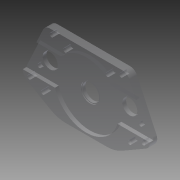
# Autodesk Inventor part: C11R1_ZP_middle wheel plate
Saved by Autodesk Inventor 2015 SP1 (Build 190203100, 203)
## iProperties
Created: 2016-01-16
Part Number: C11R1_ZP_middle wheel plate
Material: Polycarbonate, Clear
Document SubType Name: Modeling
Designer: Administrator
Density: 1.2 g/cm^3
Appearance: Polycarbonate - Clear
Mass: 206.575 g
Surface Area: 526.302 cm^2
Volume: 172.146 cm^3
Author: Administrator
Autodesk Inventor part; units mm, degrees
ref_plane "YZ Plane" through (0, 0, 0) normal (1, 0, 0) x (0, 1, 0)
ref_plane "XZ Plane" through (0, 0, 0) normal (0, 1, 0) x (-1, 0, 0)
sketch "Sketch1" plane through (0, 0, 0) normal (0, 0, 1) x (1, 0, 0)
  line L0 (0, 0) -> (0, 63.5)
  line L1 (0, 63.5) -> (203.2, 63.5)
  line L2 (203.2, 63.5) -> (203.2, 0)
  line L3 (0, 0) -> (203.2, 0)
  dimension "d0" = 63.5
  dimension "d1" = 203.2
  constraints: 8 end point, 2 perpendicular, 1 horizontal, 1 vertical
  measures "d0" distance of L0.start L0.end
  measures "d1" distance of L0.end L1.end
extrude "Extrusion1" add sketch "Sketch1" along normal blind 12.7
sketch "Sketch2" plane through (0, 0, 12.7) normal (0, 0, 1) x (1, 0, 0)
  line L0 (0, 63.5) -> (0, 0) projected
  line L1 (203.2, 0) -> (203.2, 63.5) projected
  line L2 (0, 57.2008) -> (203.2, 57.2008)
  line L3 (203.2, 57.2008) -> (203.2, 6.35)
  line L4 (203.2, 6.35) -> (0, 6.35)
  line L5 (0, 6.35) -> (0, 57.2008)
  line L6 (0, 63.5) -> (203.2, 63.5) projected
  line L7 (203.2, 0) -> (0, 0) projected
  dimension "d4" = 6.2992
  dimension "d5" = 6.35
  constraints: 8 end point, 2 parallel, 2 point on line, 1 horizontal, 1 perpendicular
  measures "d4" distance between parallel lines of L6 L2
  measures "d5" distance between parallel lines of L7 L4
extrude "Extrusion2" cut sketch "Sketch2" against normal blind 6.35 contours L2 L1 L4 L0
sketch "Sketch7" plane through (0, 0, 6.35) normal (0, 0, 1) x (1, 0, 0)
  line L0 (203.2, 6.35) -> (0, 6.35) projected
  line L1 (203.2, 57.2008) -> (203.2, 6.35) projected
  point P0 (0, 0)
  point P1 (101.6, 22.225)
  dimension "d19" = 15.875
  dimension "d20" = 101.6
  measures "d19" distance from line of L0 point (101.6, 22.225)
  measures "d20" distance from line of L1 point (101.6, 22.225)
hole "Hole1" at (101.6, 22.225, 6.35) direction (0, 0, -1) diameter 28.6258 end through all counterbore diameter 31.1658 counterbore depth 1.524
sketch "Sketch8" plane through (0, 0, 0) normal (0, 0, -1) x (-1, 0, 0)
  circle A0 centre (-34.2711, 35.4896) radius 17.78 projected
  circle A1 centre (-34.2711, 35.4896) radius 17.78 projected
  circle A2 centre (-34.2711, 35.4896) radius 17.78 projected
  line L0 (-203.2, 63.5) -> (-203.2, 0) projected
  point P0 (0, 0)
  point P1 (-168.9289, 35.4896)
  dimension "d28" = 34.2711
  measures "d28" distance from line of L0 point (-168.929, 35.49)
hole "Hole2" at (168.9289, 35.4896, 0) at (34.2711, 35.4896, 0) direction (0, 0, 1) diameter 25.4 end through all
sketch "Sketch10" plane through (0, 63.5, 0) normal (0, 1, 0) x (1, 0, 0)
  line L0 (0, -12.7) -> (203.2, -12.7)
  line L1 (203.2, -12.7) -> (203.2, 0)
  line L2 (203.2, 0) -> (0, 0)
  line L3 (0, 0) -> (0, -12.7)
  point P0 (0, 0)
  constraints: 8 end point, 2 parallel, 1 horizontal, 1 perpendicular
extrude "Extrusion5" add sketch "Sketch10" along normal blind 25.4
sketch "Sketch11" plane through (0, 6.35, 6.35) normal (-1, 0, 0) x (0, 0, 1)
  line L0 (0, 50.8508) -> (6.35, 50.8508) projected
  line L1 (6.35, 50.8508) -> (6.35, 82.55) projected
  line L2 (-6.35, 82.55) -> (6.35, 82.55) projected
  line L3 (-6.35, -6.35) -> (-6.35, 82.55) projected
  line L4 (6.35, 0) -> (6.35, -6.35) projected
  line L5 (6.35, 0) -> (0, 0) projected
  line L6 (0, 0) -> (0, 50.8508) projected
  line L7 (-6.35, -6.35) -> (6.35, -6.35) projected
extrude "Extrusion6" add sketch "Sketch11" along normal blind 9.525
sketch "Sketch12" plane through (203.2, 6.35, 6.35) normal (1, 0, 0) x (0, 0, -1)
  line L0 (-6.35, 50.8508) -> (0, 50.8508) projected
  line L1 (0, 50.8508) -> (0, 0) projected
  line L2 (0, 0) -> (-6.35, 0) projected
  line L3 (-6.35, -6.35) -> (-6.35, 0) projected
  line L4 (6.35, 82.55) -> (6.35, -6.35) projected
  line L5 (-6.35, 82.55) -> (6.35, 82.55) projected
  line L6 (-6.35, 50.8508) -> (-6.35, 82.55) projected
  line L7 (6.35, -6.35) -> (-6.35, -6.35) projected
extrude "Extrusion7" add sketch "Sketch12" along normal blind 9.525
sketch "Sketch15" plane through (0, 0, 0) normal (0, 0, -1) x (-1, 0, 0)
  circle A0 centre (-168.9289, 35.4896) radius 12.7 projected
  circle A1 centre (-34.2711, 35.4896) radius 12.7 projected
  circle A2 centre (-101.6, 22.225) radius 15.5829 projected
  line L0 (9.525, 57.2008) -> (-212.725, 57.2008) projected
  line L1 (9.525, 6.35) -> (9.525, 57.2008) projected
  line L2 (-212.725, 6.35) -> (9.525, 6.35) projected
  line L3 (-212.725, 57.2008) -> (-212.725, 6.35) projected
  line L4 (9.525, 0) -> (-41.3784, -29.3891)
  circle A3 centre (-168.9289, 35.4896) radius 12.7 projected
  circle A4 centre (-34.2711, 35.4896) radius 12.7 projected
  circle A5 centre (-101.6, 22.225) radius 14.3129 projected
  line L5 (9.525, 88.9) -> (-212.725, 88.9) projected
  line L6 (-212.725, 0) -> (-212.725, 88.9) projected
  line L7 (-212.725, 0) -> (9.525, 0) projected
  line L8 (9.525, 88.9) -> (9.525, 0) projected
  line L9 (-66.7784, -36.195) -> (-136.4216, -36.195)
  line L10 (-212.725, 0) -> (-161.8216, -29.3891)
  arc A6 (-161.8216, -29.3891) -> (-136.4216, -36.195) centre (-136.4216, 14.605) ccw
  arc A7 (-66.7784, -36.195) -> (-41.3784, -29.3891) centre (-66.7784, 14.605) ccw
  point P0 (0, 0)
  dimension "d45" = 30
  dimension "d46" = 30
  dimension "d47" = 50.8
  dimension "d48" = 58.42
  dimension "d49" = 50.8
  constraints: 6 end point, 4 point on circle, 4 tangent, 2 centre point, 1 horizontal
  measures "d45" angle of L7 L4
  measures "d46" angle of L7 L10
  measures "d47" radius of A6
  measures "d48" distance from line of L9 A2.centre
  measures "d49" radius of A7
extrude "Extrusion9" add sketch "Sketch15" against normal blind 12.7 contours L4 A7 L9 A6 L10 L7
ref_plane "Work Plane1" through (0, 88.9, 12.7) normal (0, 0, 1) x (-1, 0, 0)
sketch "Sketch16" plane through (0, 88.9, 12.7) normal (0, 0, 1) x (-1, 0, 0)
  circle A0 centre (-101.6, 66.675) radius 15.5829 projected
  circle A1 centre (-101.6, 66.675) radius 14.3129 projected
  circle A2 centre (-101.6, 66.675) radius 55.245
  point P0 (0, 88.9)
  dimension "d52" = 110.49
  constraints: 1 centre point, 1 coincident
  measures "d52" diameter of A2
extrude "Extrusion10" cut sketch "Sketch16" against normal blind 6.35 contours A2
fillet "Fillet1" radius 12.7 2 edges at (-9.525, 88.9, 6.35) (212.725, 88.9, 6.35)
sketch "Sketch18" plane through (0, 0, 0) normal (0, 0, -1) x (-1, 0, 0)
  line L0 (55.6789, 19.6749) -> (-24.8919, -17.8959) projected
  arc A0 (-32.9559, -17.0915) -> (-24.8919, -17.8959) centre (-28.2464, -10.702) ccw projected
  line L1 (-32.9559, -17.0915) -> (-58.9371, 2.0584) projected
  arc A1 (-75.7697, 38.156) -> (-58.9371, 2.0584) centre (-34.2596, 35.5391) ccw projected
  line L2 (-75.7697, 38.156) -> (-73.739, 70.3681) projected
  arc A2 (-69.1717, 77.0625) -> (-73.739, 70.3681) centre (-65.8172, 69.8687) ccw projected
  line L3 (-69.1717, 77.0625) -> (11.399, 114.6333) projected
  arc A3 (21.9474, 110.794) -> (11.399, 114.6333) centre (14.7536, 107.4395) ccw projected
  line L4 (21.9474, 110.794) -> (59.5181, 30.2233) projected
  arc A4 (55.6789, 19.6749) -> (59.5181, 30.2233) centre (52.3243, 26.8687) ccw projected
  circle A5 centre (7.2265, 11.1552) radius 4.7625 projected
  circle A6 centre (14.1519, 58.1138) radius 15.0939 projected
  circle A7 centre (23.7563, 91.8143) radius 4.7625 projected
  line L5 (51.6814, 19.5205) -> (45.6391, 23.7513) projected
  line L6 (58.3667, 22.6378) -> (51.6814, 19.5205) projected
  line L7 (59.0096, 29.9861) -> (58.3667, 22.6378) projected
  line L8 (52.9672, 34.217) -> (59.0096, 29.9861) projected
  line L9 (46.282, 31.0996) -> (52.9672, 34.217) projected
  line L10 (45.6391, 23.7513) -> (46.282, 31.0996) projected
  circle A8 centre (46.1416, 43.8088) radius 4.7625 projected
  circle A9 centre (-34.2596, 35.5391) radius 17.4625 projected
  line L11 (-4.5833, 7.3807) -> (1.459, 3.1498) projected
  line L12 (-11.2686, 4.2634) -> (-4.5833, 7.3807) projected
  line L13 (-11.9115, -3.0849) -> (-11.2686, 4.2634) projected
  line L14 (-5.8691, -7.3158) -> (-11.9115, -3.0849) projected
  line L15 (0.8161, -4.1984) -> (-5.8691, -7.3158) projected
  line L16 (1.459, 3.1498) -> (0.8161, -4.1984) projected
  line L17 (-42.1541, 87.9515) -> (-36.1117, 83.7206) projected
  line L18 (-48.8393, 84.8341) -> (-42.1541, 87.9515) projected
  line L19 (-49.4822, 77.4858) -> (-48.8393, 84.8341) projected
  line L20 (-43.4399, 73.255) -> (-49.4822, 77.4858) projected
  line L21 (-36.7546, 76.3723) -> (-43.4399, 73.255) projected
  line L22 (-36.1117, 83.7206) -> (-36.7546, 76.3723) projected
  line L23 (-27.6035, -3.3538) -> (-21.5612, -7.5847) projected
  line L24 (-34.2888, -6.4711) -> (-27.6035, -3.3538) projected
  line L25 (-34.9317, -13.8194) -> (-34.2888, -6.4711) projected
  line L26 (-28.8893, -18.0503) -> (-34.9317, -13.8194) projected
  line L27 (-22.2041, -14.9329) -> (-28.8893, -18.0503) projected
  line L28 (-21.5612, -7.5847) -> (-22.2041, -14.9329) projected
  line L29 (-65.1743, 77.217) -> (-59.132, 72.9861) projected
  line L30 (-71.8595, 74.0996) -> (-65.1743, 77.217) projected
  line L31 (-72.5024, 66.7513) -> (-71.8595, 74.0996) projected
  line L32 (-66.4601, 62.5204) -> (-72.5024, 66.7513) projected
  line L33 (-59.7749, 65.6378) -> (-66.4601, 62.5204) projected
  line L34 (-59.132, 72.9861) -> (-59.7749, 65.6378) projected
  circle A10 centre (-26.272, 82.993) radius 4.7625 projected
  circle A11 centre (-19.7768, 91.3377) radius 4.064 projected
  line L35 (8.0683, 104.3221) -> (8.7112, 111.6704) projected
  line L36 (14.1107, 100.0912) -> (8.0683, 104.3221) projected
  line L37 (20.7959, 103.2086) -> (14.1107, 100.0912) projected
  line L38 (21.4388, 110.5569) -> (20.7959, 103.2086) projected
  line L39 (15.3965, 114.7878) -> (21.4388, 110.5569) projected
  line L40 (8.7112, 111.6704) -> (15.3965, 114.7878) projected
  circle A12 centre (17.794, 10.767) radius 4.064 projected
  line L41 (-101.6, -72.6306) -> (-101.6, 117.8056)
  line L42 (-212.725, 0) -> (-212.725, 76.2) projected
  point P0 (0, 0)
  point P1 (-42.7592, 80.5977)
  point P2 (-5.1906, 0.002)
  point P3 (-174.9536, -10.702)
  point P4 (-137.3828, 69.8687)
  point P5 (-160.4408, 80.5977)
  point P6 (-198.0094, 0.002)
  dimension "d56" = 6.35
  dimension "d58" = 7.3787
  dimension "d66" = 111.125
  dimension "d73" = 6.35
  dimension "d75" = 7.3787
  constraints: 4 symmetric about line, 2 end point, 1 vertical
  measures "d56" distance from line of L16 point (-5.191, 0.002)
  measures "d58" vertical distance of L11.start point (-5.191, 0.002)
  measures "d66" distance between parallel lines of L42 L41
  measures "d73" distance from line of L22 point (-42.759, 80.598)
  measures "d75" distance of L17.start point (-42.759, 80.598)
hole "Hole3" at (42.7592, 80.5977, 0) at (5.1906, 0.002, 0) at (65.8172, 69.8687, 0) at (28.2464, -10.702, 0) at (160.4408, 80.5977, 0) at (137.3828, 69.8687, 0) at (174.9536, -10.702, 0) at (198.0094, 0.002, 0) direction (0, 0, 1) diameter 6.604 end through all clearance for "Hex Head Bolt" size "1/4" standard "Ansi Unified Screw Threads"
sketch "Sketch19" plane through (0, 0, 0) normal (0, 0, -1) x (-1, 0, 0)
  line L0 (-235.9962, 172.5258) -> (-132.2749, 172.5258)
  line L1 (-235.9962, -49.9053) -> (-235.9962, 172.5258)
  line L2 (-132.2749, 172.5258) -> (-235.9962, -49.9053)
  line L3 (-101.6, 179.9311) -> (-101.6, -67.571)
  circle A0 centre (-101.6, 22.225) radius 14.3129 projected
  line L4 (32.7962, 172.5258) -> (-70.9251, 172.5258)
  line L5 (32.7962, -49.9053) -> (32.7962, 172.5258)
  line L6 (-70.9251, 172.5258) -> (32.7962, -49.9053)
  point P0 (0, 0)
  point P1 (-212.725, 0)
  dimension "d69" = 25
  constraints: 14 end point, 3 symmetric about line, 2 point on line, 1 horizontal, 1 vertical
  measures "d69" angle of L1 L2
extrude "Extrusion11" cut sketch "Sketch19" against normal blind 25.4 contours L0 L2 L1 | L5 L6 L4
fillet "Fillet2" radius 12.7 4 edges at (171.2702, 88.9, 6.35) (212.725, 0, 6.35) (-9.525, 0, 6.35) (31.9298, 88.9, 6.35)
sketch "Sketch20" plane through (0, 0, 6.35) normal (0, 0, 1) x (1, 0, 0)
  arc A0 (-4.6068, 10.5471) -> (-5.7427, 6.35) centre (6.9033, 5.1798) ccw projected
  line L0 (48.685, 6.35) -> (-5.7427, 6.35) projected
  arc A1 (48.685, 6.35) -> (154.515, 6.35) centre (101.6, 22.225) ccw projected
  line L1 (208.9427, 6.35) -> (154.515, 6.35) projected
  arc A2 (208.9427, 6.35) -> (207.8068, 10.5471) centre (196.2967, 5.1798) ccw projected
  line L2 (207.8068, 10.5471) -> (186.0518, 57.2008) projected
  line L3 (144.3633, 57.2008) -> (186.0518, 57.2008) projected
  arc A3 (144.3633, 57.2008) -> (58.8367, 57.2008) centre (101.6, 22.225) ccw projected
  line L4 (17.1482, 57.2008) -> (58.8367, 57.2008) projected
  line L5 (17.1482, 57.2008) -> (-4.6068, 10.5471) projected
  circle A4 centre (34.2711, 35.4896) radius 12.7 projected
  circle A5 centre (101.6, 22.225) radius 15.5829 projected
  circle A6 centre (168.9289, 35.4896) radius 12.7 projected
  circle A7 centre (198.0094, 0.002) radius 3.302 projected
  circle A8 centre (28.2464, -10.702) radius 3.302 projected
  circle A9 centre (5.1906, 0.002) radius 3.302 projected
  circle A10 centre (174.9536, -10.702) radius 3.302 projected
  arc A11 (-5.7427, 6.35) -> (0.5533, -5.8187) centre (6.9033, 5.1798) ccw projected
  line L6 (0.5533, -5.8187) -> (41.3784, -29.3891) projected
  arc A12 (41.3784, -29.3891) -> (66.7784, -36.195) centre (66.7784, 14.605) ccw projected
  line L7 (66.7784, -36.195) -> (136.4216, -36.195) projected
  arc A13 (136.4216, -36.195) -> (161.8216, -29.3891) centre (136.4216, 14.605) ccw projected
  line L8 (161.8216, -29.3891) -> (202.6467, -5.8187) projected
  arc A14 (202.6467, -5.8187) -> (208.9427, 6.35) centre (196.2967, 5.1798) ccw projected
  line L9 (154.515, 6.35) -> (208.9427, 6.35) projected
  arc A15 (48.685, 6.35) -> (154.515, 6.35) centre (101.6, 22.225) ccw projected
  line L10 (-5.7427, 6.35) -> (48.685, 6.35) projected
  arc A16 (40.0205, 88.9) -> (28.5104, 81.5673) centre (40.0205, 76.2) ccw projected
  line L11 (28.5104, 81.5673) -> (17.1482, 57.2008) projected
  line L12 (17.1482, 57.2008) -> (58.8367, 57.2008) projected
  arc A17 (144.3633, 57.2008) -> (58.8367, 57.2008) centre (101.6, 22.225) ccw projected
  line L13 (144.3633, 57.2008) -> (186.0518, 57.2008) projected
  line L14 (186.0518, 57.2008) -> (174.6896, 81.5673) projected
  arc A18 (174.6896, 81.5673) -> (163.1795, 88.9) centre (163.1795, 76.2) ccw projected
  line L15 (163.1795, 88.9) -> (40.0205, 88.9) projected
  circle A19 centre (137.3828, 69.8687) radius 3.302 projected
  circle A20 centre (42.7592, 80.5977) radius 3.302 projected
  circle A21 centre (65.8172, 69.8687) radius 3.302 projected
  circle A22 centre (160.4408, 80.5977) radius 3.302 projected
  point P0 (0, 0)
  point P1 (187.325, 19.05)
  point P2 (15.875, 19.05)
  dimension "d76" = 12.7
  dimension "d77" = 85.725
  dimension "d78" = 85.725
  dimension "d79" = 12.7
  measures "d76" distance from line of L1 point (187.325, 19.05)
  measures "d77" horizontal distance of A1.centre point (187.325, 19.05)
  measures "d78" horizontal distance of A1.centre point (15.875, 19.05)
  measures "d79" distance from line of point (15.875, 19.05) L0
hole "Hole4" at (187.325, 19.05, 6.35) at (15.875, 19.05, 6.35) direction (0, 0, -1) diameter 6.604 end through all clearance for "Flat Head Machine Screw (82)" size "1/4" standard "Ansi Unified Screw Threads"
sketch "Sketch21" plane through (0, 0, 6.35) normal (0, 0, 1) x (1, 0, 0)
  circle A0 centre (187.325, 19.05) radius 3.302 projected
  circle A1 centre (15.875, 19.05) radius 3.302 projected
  arc A2 (-4.6068, 10.5471) -> (-5.7427, 6.35) centre (6.9033, 5.1798) ccw projected
  line L0 (48.685, 6.35) -> (-5.7427, 6.35) projected
  arc A3 (48.685, 6.35) -> (154.515, 6.35) centre (101.6, 22.225) ccw projected
  line L1 (208.9427, 6.35) -> (154.515, 6.35) projected
  arc A4 (208.9427, 6.35) -> (207.8068, 10.5471) centre (196.2967, 5.1798) ccw projected
  line L2 (207.8068, 10.5471) -> (186.0518, 57.2008) projected
  line L3 (144.3633, 57.2008) -> (186.0518, 57.2008) projected
  arc A5 (144.3633, 57.2008) -> (58.8367, 57.2008) centre (101.6, 22.225) ccw projected
  line L4 (17.1482, 57.2008) -> (58.8367, 57.2008) projected
  line L5 (17.1482, 57.2008) -> (-4.6068, 10.5471) projected
  circle A6 centre (34.2711, 35.4896) radius 12.7 projected
  circle A7 centre (101.6, 22.225) radius 15.5829 projected
  circle A8 centre (168.9289, 35.4896) radius 12.7 projected
  arc A9 (40.0205, 88.9) -> (28.5104, 81.5673) centre (40.0205, 76.2) ccw projected
  line L6 (28.5104, 81.5673) -> (17.1482, 57.2008) projected
  line L7 (17.1482, 57.2008) -> (58.8367, 57.2008) projected
  arc A10 (144.3633, 57.2008) -> (58.8367, 57.2008) centre (101.6, 22.225) ccw projected
  line L8 (144.3633, 57.2008) -> (186.0518, 57.2008) projected
  line L9 (186.0518, 57.2008) -> (174.6896, 81.5673) projected
  arc A11 (174.6896, 81.5673) -> (163.1795, 88.9) centre (163.1795, 76.2) ccw projected
  line L10 (163.1795, 88.9) -> (40.0205, 88.9) projected
  circle A12 centre (137.3828, 69.8687) radius 3.302 projected
  circle A13 centre (42.7592, 80.5977) radius 3.302 projected
  circle A14 centre (65.8172, 69.8687) radius 3.302 projected
  circle A15 centre (160.4408, 80.5977) radius 3.302 projected
  circle A16 centre (198.0094, 0.002) radius 3.302 projected
  circle A17 centre (28.2464, -10.702) radius 3.302 projected
  circle A18 centre (5.1906, 0.002) radius 3.302 projected
  circle A19 centre (174.9536, -10.702) radius 3.302 projected
  arc A20 (-5.7427, 6.35) -> (0.5533, -5.8187) centre (6.9033, 5.1798) ccw projected
  line L11 (0.5533, -5.8187) -> (41.3784, -29.3891) projected
  arc A21 (41.3784, -29.3891) -> (66.7784, -36.195) centre (66.7784, 14.605) ccw projected
  line L12 (66.7784, -36.195) -> (136.4216, -36.195) projected
  arc A22 (136.4216, -36.195) -> (161.8216, -29.3891) centre (136.4216, 14.605) ccw projected
  line L13 (161.8216, -29.3891) -> (202.6467, -5.8187) projected
  arc A23 (202.6467, -5.8187) -> (208.9427, 6.35) centre (196.2967, 5.1798) ccw projected
  line L14 (154.515, 6.35) -> (208.9427, 6.35) projected
  arc A24 (48.685, 6.35) -> (154.515, 6.35) centre (101.6, 22.225) ccw projected
  line L15 (-5.7427, 6.35) -> (48.685, 6.35) projected
  circle A25 centre (101.6, 22.225) radius 14.3129 projected
  point P0 (0, 0)
body "Solid1"
